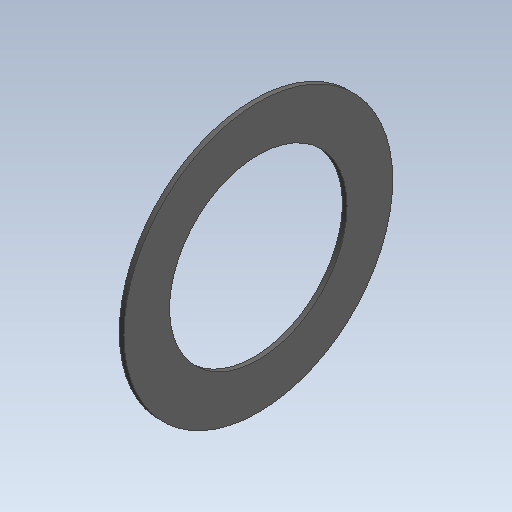
# Autodesk Inventor part: MF126ZZ Shield1
Saved by Autodesk Inventor 2020.2 (Build 242310000, 310)
## iProperties
Part Number: MF126ZZ Shield1
Material: 一般
Catalog Web Link: www.cadenas.de
Description: shielded_type_zz_zzs_S1-
Vendor: NSK_RB
Document SubType Name: Modeling
Designer: partserver
Manufacturer: NSK_RB
Mass: 0.00985689 g
Surface Area: 1.15852 cm^2
Volume: 0.00985689 cm^3
Density: 1 g/cm^3
Appearance: PSOLRGB-128-128-128
Category: PARTsolutions
Company: NSK_RB
PSOL_IDENT_0: {$CADENAS_DATA\23d-libs\nsk_rb\roller_bearings\deep_groove_bb\exstra_small_miniatur_bb\metric_design
PSOL_IDENT_1: _with_flange\shielded_type_zz_zzs_s1_1a.prj},188 {VTYP=3D},{NB=MF126ZZ Shield1},{LINA=MF126ZZ Shield
PSOL_IDENT_2: 1},{NN=shielded_type_zz_zzs_S1},{DATE=10.04.2020 04:57:39},{GEOMDATE=04.01.2008 00:00:00},{VERSION=}
PSOL_IDENT_3: ,{LINEID=570},{WBVAR=},{WBNUMERIC=}  {NB=MF126ZZ Shield1},{LINA=MF126ZZ Shield1},{KT=DUMMY},{IDNR=},
PSOL_IDENT_4: {STAN=},{ORDER=MF126ZZ},{SD=6.0},{X=6.0},{D=12},{DD=12},{DD1=0.0},{D2=13.6},{DD2=13.6},{B=0.0},{B1=4
PSOL_IDENT_5: .0},{CC1=0.0},{C2=0.8},{CC2=0.8},{R=0.00},{R1=0.15},{DI1=7.73},{DI2=7.20},{SDE1=10.19},{SDE2=10.90},
PSOL_IDENT_6: {CR1=715},{COR1=292},{CR2=73},{COR2=30.0},{LG=43000},{LO=50000},{DA=0.0},{DB=7.2},{RA=0.00},{RB=0.15
PSOL_IDENT_7: },{MASS=1.94},{SC=1}
NB: MF126ZZ Shield1
NN: shielded_type_zz_zzs_S1
NBSYN: $ORDER. Shield1
LINA: MF126ZZ Shield1
CATALOG: NSK Rolling Bearing
ORDER: MF126ZZ
SD: 6
X: 6
D: 12
DD: 12
DD1: 0
D2: 13.6
DD2: 13.6
B: 0
B1: 4
CC1: 0
C2: 0.8
CC2: 0.8
R: 0
R1: 0.15
DI1: 7.73
DI2: 7.2
SDE1: 10.19
SDE2: 10.9
CR1: 715
COR1: 292
CR2: 73
COR2: 30
LG: 43000
LO: 50000
DA: 0
DB: 7.2
RA: 0
RB: 0.15
MASS: 1.94
SC: 1
SUPPLIER: NSK_RB
ARTICLENO: MF126ZZ Shield1
BOMINFO: MF126ZZ Shield1
CREATOR: CADENAS GmbH
Title: MF126ZZ Shield1
Author: Cadenas PARTsolutions
Autodesk Inventor part; units mm, degrees
sketch "Sketch_1" plane through (0, 0, 0) normal (0, 0, 1) x (1, 0, 0)
  line L0 (0.4374, 0) -> (0.25, 0)
  line L1 (0.25, 3.6) -> (0.4374, 3.6)
  line L2 (0.4374, 3.6) -> (0.4374, 5.45)
  line L3 (0.4374, 5.45) -> (0.25, 5.45)
  line L4 (0.25, 5.45) -> (0.25, 3.6)
  constraints: 10 end point
revolve "Revolution1" add sketch "Sketch_1" angle 360 about axis through (0.4374, 0, 0) along (1, 0, 0)
ref_plane "ip_st_1_XY" through (0.25, 0, 0) normal (-1, 0, 0) x (0, 0, -1)
ref_plane "ip_st_1_YZ" through (0.25, 0, 0) normal (0, 0, -1) x (0, -1, 0)
ref_plane "ip_st_1_ZX" through (0.25, 0, 0) normal (0, -1, 0) x (-1, 0, 0)
body "Solid1"
